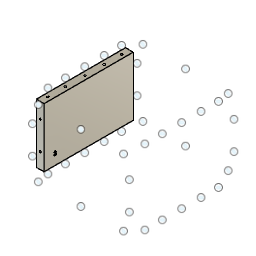
CAD_File 4 (Autodesk Fusion 360 design; units mm, degrees)
Autodesk Fusion 360 part; units mm, degrees
sketch "Sketch1" plane through (0, 0, -20) normal (0, 0, -1) x (1, 0, 0)
  circle A0 centre (15, 75) radius 1.5
  circle A1 centre (-15, 75) radius 1.5
  circle A2 centre (15, 45) radius 1.5
  circle A3 centre (-15, 45) radius 1.5
  circle A4 centre (0, 60) radius 14
  line L0 (-135, -115) -> (135, -115)
  line L1 (135, -115) -> (135, 115)
  line L2 (135, 115) -> (-135, 115)
  line L3 (-135, 115) -> (-135, -115)
  line L4 (-135, 115) -> (-115, 115)
  line L5 (-115, 115) -> (-115, -115)
  line L6 (-115, -115) -> (-135, -115)
  line L7 (-135, -115) -> (-135, 115)
  dimension "d481" = 20
  constraint horizontal L4
  constraint vertical L5
  constraint horizontal L6
  constraint vertical L7
  constraint coincident L2.end L3.start
  measures "d481" distance of L2.end L4.end
extrude "Extrude1" add sketch "Sketch1" along normal blind 152.35 contours L0 L2 L3 L4 L5 L6 L7
sketch "sketch 1206" plane through (0, 0, 0) normal (0, 0, 1) x (-1, 0, 0)
  circle A0 centre (-125, 0) radius 3
  circle A1 centre (125, 95) radius 3
  circle A2 centre (125, -95) radius 3
  circle A3 centre (125, 0) radius 3
  circle A4 centre (-125, 95) radius 3
  circle A5 centre (-125, -95) radius 3
extrude "Extrude2" cut sketch "sketch 1206" against normal blind 40
sketch "sketch 1239" plane through (0, 0, 0) normal (0, 0, 1) x (-1, 0, 0)
  circle A0 centre (-125, 50) radius 3
  circle A1 centre (125, -50) radius 3
  circle A2 centre (125, 50) radius 3
  circle A3 centre (-125, -50) radius 3
extrude "Extrude3" cut sketch "sketch 1239" against normal blind 35
sketch "sketch 1263" plane through (0, 0, -192.35) normal (0, 0, -1) x (1, 0, 0)
  circle A0 centre (125, 0) radius 3
  circle A1 centre (-125, 95) radius 3
  circle A2 centre (-125, -95) radius 3
  circle A3 centre (-125, 0) radius 3
  circle A4 centre (125, 95) radius 3
  circle A5 centre (125, -95) radius 3
extrude "Extrude4" cut sketch "sketch 1263" against normal blind 40
sketch "sketch 1295" plane through (0, 0, -192.35) normal (0, 0, -1) x (1, 0, 0)
  circle A0 centre (-125, -50) radius 3
  circle A1 centre (125, -50) radius 3
  circle A2 centre (125, 50) radius 3
  circle A3 centre (-125, 50) radius 3
extrude "Extrude5" cut sketch "sketch 1295" against normal blind 35
sketch "sketch 1319" plane through (0, 135, 0) normal (0, 1, 0) x (-1, 0, 0)
  circle A0 centre (-110, -182.35) radius 3
  circle A1 centre (110, -182.35) radius 3
  circle A2 centre (125, -60) radius 3
  circle A3 centre (0, -10) radius 3
  circle A4 centre (-125, -60) radius 3
  circle A5 centre (-110, -10) radius 3
  circle A6 centre (110, -10) radius 3
  circle A7 centre (125, -132.35) radius 3
  circle A8 centre (0, -182.35) radius 3
  circle A9 centre (-125, -132.35) radius 3
extrude "Extrude6" cut sketch "sketch 1319" against normal blind 40
sketch "sketch 1367" plane through (0, -135, 0) normal (0, -1, 0) x (1, 0, 0)
  circle A0 centre (-110, -182.35) radius 3
  circle A1 centre (110, -182.35) radius 3
  circle A2 centre (125, -60) radius 3
  circle A3 centre (0, -10) radius 3
  circle A4 centre (-125, -60) radius 3
  circle A5 centre (-110, -10) radius 3
  circle A6 centre (110, -10) radius 3
  circle A7 centre (125, -132.35) radius 3
  circle A8 centre (0, -182.35) radius 3
  circle A9 centre (-125, -132.35) radius 3
extrude "Extrude7" cut sketch "sketch 1367" against normal blind 40
thread "Thread1" "ISO Metric profile 6.0 M6x1 6H" major diameter 6.147 minor diameter 5.035 pitch 1 angle 60 resizes the face on face at (-122.3653, 93.5652, -165.6833) on face at (-127.0947, 108.3333, -130.2024) on face at (-126.9851, -101.6667, -62.2493) on face at (-126.2339, -2.7345, -165.6833) on face at (-122.3653, -96.4348, -165.6833) on face at (-122.9053, -108.3333, -130.2024) on face at (-123.0149, 101.6667, -62.2493) on face at (-127.6347, -96.4348, -26.6667) on face at (-123.7661, -2.7345, -26.6667) on face at (-127.6347, 93.5652, -26.6667)
sketch "Sketch3" plane through (-115, 0, 0) normal (1, 0, 0) x (0, 1, 0)
  line L0 (115, -20) -> (-115, -20)
  line L1 (-115, -20) -> (-115, -172.35)
  line L2 (-115, -172.35) -> (115, -172.35)
  line L3 (115, -172.35) -> (115, -20)
  line L4 (-83.3765, -148.8199) -> (-83.3765, -150)
  line L5 (-83.3765, -150) -> (-89.9864, -150)
  spline S0 degree 2 poles (-89.9864, -150) (-90, -149.5566) (-89.8431, -149.1473) knots 0 0 0 1 1 1
  spline S1 degree 2 poles (-89.8431, -149.1473) (-89.5907, -148.472) (-89.0348, -147.8172) knots 0 0 0 1 1 1
  spline S2 degree 2 poles (-89.0348, -147.8172) (-88.4789, -147.1623) (-87.4284, -146.3029) knots 0 0 0 1 1 1
  spline S3 degree 2 poles (-87.4284, -146.3029) (-85.7981, -144.9659) (-85.2251, -144.1849) knots 0 0 0 1 1 1
  spline S4 degree 2 poles (-85.2251, -144.1849) (-84.6521, -143.4038) (-84.6521, -142.708) knots 0 0 0 1 1 1
  spline S5 degree 2 poles (-84.6521, -142.708) (-84.6521, -141.9782) (-85.1739, -141.4768) knots 0 0 0 1 1 1
  spline S6 degree 2 poles (-85.1739, -141.4768) (-85.6958, -140.9754) (-86.5348, -140.9754) knots 0 0 0 1 1 1
  spline S7 degree 2 poles (-86.5348, -140.9754) (-87.4216, -140.9754) (-87.9536, -141.5075) knots 0 0 0 1 1 1
  spline S8 degree 2 poles (-87.9536, -141.5075) (-88.4857, -142.0396) (-88.4925, -142.9809) knots 0 0 0 1 1 1
  line L6 (-88.4925, -142.9809) -> (-89.7544, -142.8513)
  spline S9 degree 2 poles (-89.7544, -142.8513) (-89.6248, -141.4393) (-88.779, -140.6992) knots 0 0 0 1 1 1
  spline S10 degree 2 poles (-88.779, -140.6992) (-87.9332, -139.9591) (-86.5075, -139.9591) knots 0 0 0 1 1 1
  spline S11 degree 2 poles (-86.5075, -139.9591) (-85.0682, -139.9591) (-84.2292, -140.7572) knots 0 0 0 1 1 1
  spline S12 degree 2 poles (-84.2292, -140.7572) (-83.3902, -141.5553) (-83.3902, -142.7353) knots 0 0 0 1 1 1
  spline S13 degree 2 poles (-83.3902, -142.7353) (-83.3902, -143.3356) (-83.6357, -143.9154) knots 0 0 0 1 1 1
  spline S14 degree 2 poles (-83.6357, -143.9154) (-83.8813, -144.4952) (-84.4509, -145.1364) knots 0 0 0 1 1 1
  spline S15 degree 2 poles (-84.4509, -145.1364) (-85.0205, -145.7776) (-86.3438, -146.8963) knots 0 0 0 1 1 1
  spline S16 degree 2 poles (-86.3438, -146.8963) (-87.4488, -147.824) (-87.7626, -148.1548) knots 0 0 0 1 1 1
  spline S17 degree 2 poles (-87.7626, -148.1548) (-88.0764, -148.4857) (-88.281, -148.8199) knots 0 0 0 1 1 1
  line L7 (-88.281, -148.8199) -> (-83.3765, -148.8199)
extrude "Extrude9" cut sketch "Sketch3" against normal blind 0.2 contours L4 L5 S0 S1 S2 S3 S4 S5 S6 S7 S8 L6 S9 S10 S11 S12 S13 S14 S15 S16 S17 L7
